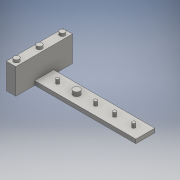
# Autodesk Inventor part: Kroller Holder2
Saved by Autodesk Inventor 2016 (Build 200138000, 138)
## iProperties
Created: 2018-03-02
Part Number: Kroller Holder2
Material: Generic
Document SubType Name: Modeling
Designer: Simon
Density: 1 g/cm^3
Appearance: Default
Author: Simon
Autodesk Inventor part; units mm, degrees
ref_plane "YZ Plane" through (0, 0, 0) normal (1, 0, 0) x (0, 1, 0)
ref_plane "XZ Plane" through (0, 0, 0) normal (0, 1, 0) x (-1, 0, 0)
ref_plane "XY Plane" through (0, 0, 0) normal (0, 0, 1) x (1, 0, 0)
sketch "Sketch1" plane through (0, 0, 0) normal (0, 0, 1) x (1, 0, 0)
  line L0 (0, 0) -> (70, 0)
  line L1 (70, 0) -> (70, 14)
  line L2 (70, 14) -> (0, 14)
  line L3 (0, 14) -> (0, 0)
  dimension "d0" = 70
  dimension "d1" = 14
  constraints: 8 end point, 2 parallel, 1 horizontal, 1 perpendicular
  measures "d0" distance of L2.end L1.end
  measures "d1" distance of L1.end L0.end
extrude "Extrusion1" add sketch "Sketch1" along normal blind 1
sketch "Sketch2" plane through (0, 0, 1) normal (0, 0, 1) x (1, 0, 0)
  line L0 (70, 14) -> (0, 14) projected
  line L1 (0, 14) -> (0, 0) projected
  circle A0 centre (7, 7) radius 1.225
  circle A1 centre (35.2, 7) radius 1.225
  dimension "d5" = 70
  dimension "d6" = 14
  dimension "d9" = 2.45
  dimension "d10" = 2.45
  dimension "d32" = 28.2
  constraints: 2 centre point
  measures "d5" distance of L0.start L0.end
  measures "d6" distance of L0.end L1.end
  measures "d9" diameter of A0
  measures "d10" diameter of A1
  measures "d32" distance of A1.centre A0.centre
extrude "Extrusion5" add sketch "Sketch2" along normal blind 3
sketch "Sketch4" plane through (0, 0, 1) normal (0, 0, 1) x (1, 0, 0)
  circle A0 centre (21.1, 7) radius 2.5
  line L0 (0, 0) -> (70, 0) projected
  line L1 (0, 14) -> (0, 0) projected
  circle A1 centre (7, 7) radius 1.225 projected
  point P0 (6, 0)
  point P1 (64, 0)
  point P2 (0, 8)
  point P3 (0, 6)
  dimension "d25" = 5
  dimension "d26" = 7
  dimension "d29" = 14.1
  constraints: 1 centre point
  measures "d25" diameter of A0
  measures "d26" distance from line of L0 A0.centre
  measures "d29" distance of A1.centre A0.centre
extrude "Extrusion6" add sketch "Sketch4" along normal blind 3 contours A0
sketch "Sketch5" plane through (0, 0, 1) normal (0, 0, 1) x (1, 0, 0)
  circle A0 centre (35.2, 7) radius 1.225 projected
  circle A1 centre (49.3, 7) radius 1.225
  point P0 (0, 0)
  dimension "d34" = 14.1
  constraints: 1 centre point
  measures "d34" distance of A1.centre A0.centre
extrude "Extrusion7" add sketch "Sketch5" along normal blind 3 contours A1
pattern_linear "Rectangular Pattern2" count 2 spacing 14.1 along (1, 0, 0) of "Extrusion7"
sketch "Sketch6" plane through (0, 0, 0) normal (-1, 0, 0) x (0, 0, 1)
  line L0 (1, 0) -> (1, 14) projected
  line L1 (0, 0) -> (1, 0)
  line L2 (1, 0) -> (1, 14)
  line L3 (1, 14) -> (0, 14)
  line L4 (0, 14) -> (0, 0)
  line L5 (0, 14) -> (1, 14)
  line L6 (0, 0) -> (1, 0) projected
  line L7 (0, 0) -> (1, 0)
  constraints: 12 end point, 3 horizontal, 2 parallel, 1 perpendicular
extrude "Extrusion8" add sketch "Sketch6" along normal blind 10
sketch "Sketch7" plane through (-10, 0, 0) normal (-1, 0, 0) x (0, 0, 1)
  line L0 (0, 0) -> (1, 0) projected
  line L1 (0, 0) -> (1, 0)
  line L2 (1, 0) -> (1, -14)
  line L3 (1, -14) -> (0, -14)
  line L4 (0, -14) -> (0, 0)
  line L5 (0, 13.9913) -> (1, 13.9913)
  line L6 (1, 13.9913) -> (1, 27.9913)
  line L7 (1, 27.9913) -> (0, 27.9913)
  line L8 (0, 27.9913) -> (0, 13.9913)
  line L9 (1, 0) -> (1, 14) projected
  line L10 (0, 0) -> (0, 14) projected
  line L11 (1, 14) -> (0, 14)
  line L12 (0, 14) -> (0, 0)
  line L13 (0, 0) -> (1, 0)
  line L14 (1, 0) -> (1, 14)
  dimension "d47" = 14
  dimension "d48" = 14
  constraints: 24 end point, 6 parallel, 3 horizontal, 3 perpendicular, 2 point on line
  measures "d47" distance of L1.end L2.end
  measures "d48" distance of L6.end L5.end
extrude "Extrusion9" add sketch "Sketch7" against normal blind 7
sketch "Sketch8" plane through (0, 0, 0) normal (0, 0, -1) x (-1, 0, 0)
  line L0 (10, 27.9913) -> (10, -14) projected
  line L1 (10, 27.9913) -> (3, 27.9913)
  line L2 (3, 27.9913) -> (3, -14)
  line L3 (3, -14) -> (10, -14)
  line L4 (10, -14) -> (10, 27.9913)
  line L5 (-70, 0) -> (-70, 14) projected
  line L6 (-70, 14) -> (3, 14) projected
  line L7 (-70, 0) -> (3, 0)
  line L8 (3, 0) -> (3, 14)
  line L9 (3, 14) -> (-70, 14)
  line L10 (-70, 14) -> (-70, 0)
  point P0 (0, 0)
  constraints: 16 end point, 4 parallel, 2 horizontal, 2 perpendicular
extrude "Extrusion10" add sketch "Sketch8" along normal blind 2
sketch "Sketch9" plane through (0, 0, 1) normal (0, 0, 1) x (1, 0, 0)
  circle A0 centre (-6.5, 23.9913) radius 2
  line L0 (-3, 27.9913) -> (-3, 14) projected
  line L1 (-10, 27.9913) -> (-3, 27.9913) projected
  circle A1 centre (-6.5, 6.9913) radius 2
  circle A2 centre (-6.5, -10.0087) radius 2
  line L2 (-10, -14) -> (-3, -14) projected
  line L3 (-10, -14) -> (-10, 27.9913) projected
  point P0 (0, 0)
  dimension "d53" = 4
  dimension "d54" = 3.5
  dimension "d55" = 4
  dimension "d58" = 17
  dimension "d63" = 41.9913
  dimension "d64" = 17
  dimension "d65" = 3.9913
  constraints: 3 centre point, 1 vertical, 4 other
  measures "d53" diameter of A0
  measures "d54" distance from line of L0 A0.centre
  measures "d55" distance from line of L1 A0.centre
  measures "d58" distance of A0.centre A1.centre
  measures "d63" distance of L2.start L1.start
  measures "d64" distance of A2.centre A1.centre
  measures "d65" distance from line of L2 A2.centre
extrude "Extrusion11" add sketch "Sketch9" along normal blind 18
sketch "Sketch10" plane through (0, 0, 1) normal (0, 0, 1) x (1, 0, 0)
  line L0 (-10, -14) -> (-3, -14) projected
  line L1 (-3, 27.9913) -> (-10, 27.9913)
  line L2 (-10, 27.9913) -> (-10, -14)
  line L3 (-10, -14) -> (-3, -14)
  line L4 (-3, -14) -> (-3, 27.9913)
  point P0 (0, 0)
  constraints: 8 end point, 2 parallel, 1 coincident, 1 horizontal, 1 perpendicular
extrude "Extrusion12" add sketch "Sketch10" along normal blind 16
sketch "Sketch11" plane through (70, 0, 1) normal (1, 0, 0) x (0, 0, -1)
  line L0 (3, 0) -> (0, 0) projected
  line L1 (3, 14) -> (0, 14) projected
  line L2 (3, 0) -> (0, 0)
  line L3 (0, 0) -> (0, 14)
  line L4 (0, 14) -> (3, 14)
  line L5 (3, 14) -> (3, 0)
  point P0 (1, 0)
  constraints: 8 end point, 2 parallel, 1 horizontal, 1 perpendicular
extrude "Extrusion13" add sketch "Sketch11" along normal blind 2
body "Solid1"
